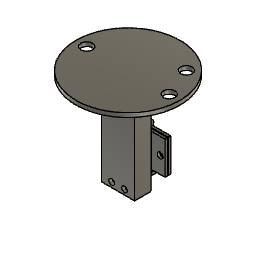
electrode_jig (Autodesk Fusion 360 design; units mm, degrees)
Autodesk Fusion 360 part; units mm, degrees
note: some values were not read from the file. Set by a fixed rule: which sketch regions a step uses.
sketch "スケッチ1" plane through (0, 0, 0) normal (0, 0, 1) x (1, 0, 0)
  circle A0 centre (0, 0) radius 31.5
  circle A1 centre (0, 0) radius 25 construction
  circle A2 centre (-25, 0) radius 3.5
  circle A3 centre (25, 0) radius 3.5
  line L0 (0, 1.75) -> (0, 22.5)
  line L1 (1.75, 0) -> (22.5, 0)
  circle A4 centre (17.6777, 17.6777) radius 3.5
  line L2 (17.6777, 17.6777) -> (0, 0) construction
  dimension "d1" = 63
  dimension "d2" = 50
  dimension "d5" = 7
  dimension "d6" = 7
  dimension "d7" = 7
  dimension "d8" = 45
  constraint coincident A0.centre A1.centre
  constraint coincident A1 A2.centre
  constraint coincident A1 A3.centre
  constraint coincident A3.centre L1
  constraint coincident A2.centre L1
  constraint coincident A1 A4.centre
  constraint coincident A4.centre L2.start
  measures "d1" diameter of A0
  measures "d2" diameter of A1
  measures "d5" diameter of A2
  measures "d6" diameter of A3
  measures "d7" diameter of A4
  measures "d8" angle of L1 L2
extrude "押し出し1" add sketch "スケッチ1" along normal blind 2.5 makes body 1
sketch "スケッチ17" plane through (0, 0, 0) normal (0, 0, -1) x (1, 0, 0)
  circle A0 centre (25, 0) radius 3.5
  circle A1 centre (-25, 0) radius 3.5
  circle A2 centre (17.6777, -17.6777) radius 3.5
  circle A3 centre (0, 0) radius 31.5
  line L0 (10, -4) -> (8, -4)
  line L1 (8, -4) -> (8, 4)
  line L2 (8, 4) -> (-8, 4)
  line L3 (-8, 4) -> (-8, -4)
  line L4 (-8, -4) -> (-10, -4)
  line L5 (-10, -4) -> (-10, 6)
  line L6 (-10, 6) -> (10, 6)
  line L7 (10, 6) -> (10, -4)
  line L8 (8, -4) -> (6, -4)
  line L9 (6, -4) -> (6, -2)
  line L10 (6, -2) -> (8, -2)
  line L11 (8, -2) -> (8, -4)
  line L12 (-8, -4) -> (-6, -4)
  line L13 (-6, -4) -> (-6, -2)
  line L14 (-6, -2) -> (-8, -2)
  line L15 (-8, -2) -> (-8, -4)
  dimension "d138" = 16
  dimension "d139" = 2
  dimension "d140" = 2
  dimension "d142" = 8
  dimension "d143" = 2
  dimension "d144" = 4
  dimension "d145" = 8
  dimension "d178" = 2
  dimension "d179" = 2
  dimension "d180" = 2
  dimension "d181" = 2
  constraint horizontal L0
  constraint perpendicular L0 L1
  constraint perpendicular L1 L2
  constraint perpendicular L2 L3
  constraint perpendicular L1 L4
  constraint perpendicular L4 L5
  constraint perpendicular L1 L6
  constraint perpendicular L6 L7
  constraint collinear L0 L4
  constraint horizontal L8
  constraint vertical L9
  constraint horizontal L10
  constraint vertical L11
  constraint horizontal L12
  constraint vertical L13
  constraint horizontal L14
  constraint vertical L15
  measures "d138" distance of L1.end L2.end
  measures "d139" distance of L3.end L4.end
  measures "d140" distance of L0.start L0.end
  measures "d142" distance of L0.end L1.end
  measures "d143" distance of L2 L6
  measures "d144" distance of A3.centre L2
  measures "d145" distance of A3.centre L3
  measures "d178" distance of L0.end L8.end
  measures "d179" distance of L8.end L9.end
  measures "d180" distance of L3.end L12.end
  measures "d181" distance of L12.end L13.end
extrude "押し出し16" add sketch "スケッチ17" along normal blind 58 contours L0 L1 L2 L3 L4 L5 L6 L7 L11 L15 | L1 L8 L9 L10 L11 | L3 L12 L13 L14 L15 bodies 1
sketch "スケッチ24" plane through (0, 0, 0) normal (0, 0, -1) x (1, 0, 0)
  line L0 (-10, -4) -> (-10, 6)
  line L1 (-10, 6) -> (10, 6)
  line L2 (10, 6) -> (10, -4)
  line L3 (10, -4) -> (6, -4)
  line L4 (6, -4) -> (6, -2)
  line L5 (6, -2) -> (8, -2)
  line L6 (8, -2) -> (8, 4)
  line L7 (8, 4) -> (-8, 4)
  line L8 (-8, 4) -> (-8, -2)
  line L9 (-8, -2) -> (-6, -2)
  line L10 (-6, -2) -> (-6, -4)
  line L11 (-6, -4) -> (-10, -4)
  circle A0 centre (17.6777, -17.6777) radius 3.5
  circle A1 centre (25, 0) radius 3.5
  circle A2 centre (-25, 0) radius 3.5
  circle A3 centre (0, 0) radius 31.5
  line L12 (-10, 6) -> (10, 6)
  line L13 (10, 6) -> (10, -4)
  line L14 (10, -4) -> (-10, -4)
  line L15 (-10, -4) -> (-10, 6)
  constraint horizontal L12
  constraint vertical L13
  constraint horizontal L14
  constraint vertical L15
  constraint coincident L2.end L3.start
  constraint coincident L0.end L1.start
extrude "押し出し24" add sketch "スケッチ24" along normal blind 5 contours L0 L1 L2 L3 L4 L5 L6 L7 L8 L9 L10 L11 L12 L13 L14 L15 | L4 L5 L6 L7 L8 L9 L10 L14 bodies 1
sketch "スケッチ19" plane through (0, 0, 0) normal (0, 0, -1) x (1, 0, 0)
  line L0 (10, 6) -> (10, -4)
  line L1 (10, -4) -> (-10, -4)
  line L2 (-10, -4) -> (-10, 6)
  line L3 (-10, 6) -> (10, 6)
  circle A0 centre (25, 0) radius 3.5
  circle A1 centre (-25, 0) radius 3.5
  circle A2 centre (17.6777, -17.6777) radius 3.5
  circle A3 centre (0, 0) radius 31.5
  circle A4 centre (0, 0) radius 2
  dimension "d152" = 4
  constraint coincident A3.centre A4.centre
  measures "d152" diameter of A4
extrude "押し出し18" add sketch "スケッチ19" along normal blind 50 contours A4 bodies 1
sketch "スケッチ20" plane through (0, 0, -50) normal (0, 0, -1) x (1, 0, 0)
  circle A0 centre (0, 0) radius 2
  line L0 (7.9, -13.5) -> (-7.9, -13.5)
  line L1 (-7.9, -13.5) -> (-7.9, 3.9)
  line L2 (-7.9, 3.9) -> (7.9, 3.9)
  line L3 (7.9, 3.9) -> (7.9, -13.5)
  line L4 (-10, -4) -> (-6, -4)
  line L5 (10, 6) -> (-10, 6)
  line L6 (-10, 6) -> (-10, -4)
  line L7 (-10, -4) -> (-6, -4)
  line L8 (-8, -2) -> (-8, 4)
  line L9 (-8, 4) -> (8, 4)
  line L10 (8, 4) -> (8, -2)
  line L11 (10, -4) -> (10, 6)
  circle A1 centre (0, -8.5) radius 3.25
  line L12 (0, 0) -> (0, -8.5) construction
  line L13 (-6, -4) -> (-6, -2)
  line L14 (-6, -2) -> (-8, -2)
  line L15 (8, -2) -> (6, -2)
  line L16 (6, -2) -> (6, -4)
  line L17 (6, -4) -> (10, -4)
  line L18 (-10, -4) -> (-6, -4)
  line L19 (-6, -4) -> (-6, -2)
  line L20 (-6, -2) -> (-8, -2)
  line L21 (-8, -2) -> (-8, 4)
  line L22 (-8, 4) -> (8, 4)
  line L23 (8, 4) -> (8, -2)
  line L24 (8, -2) -> (6, -2)
  line L25 (6, -2) -> (6, -4)
  line L26 (6, -4) -> (10, -4)
  line L27 (10, -4) -> (10, 6)
  line L28 (10, 6) -> (-10, 6)
  line L29 (-10, 6) -> (-10, -4)
  circle A2 centre (0, 0) radius 2
  line L30 (-7.9, -4.15) -> (-5.8, -4.15)
  line L31 (-5.8, -4.15) -> (-5.8, -1.85)
  line L32 (-5.8, -1.85) -> (-7.9, -1.85)
  line L33 (-7.9, -1.85) -> (-7.9, -4.15)
  line L34 (7.9, -4.15) -> (5.8, -4.15)
  line L35 (5.8, -4.15) -> (5.8, -1.85)
  line L36 (5.8, -1.85) -> (7.9, -1.85)
  line L37 (7.9, -1.85) -> (7.9, -4.15)
  dimension "d155" = 0.1
  dimension "d156" = 0.1
  dimension "d157" = 0.1
  dimension "d173" = 6.5
  dimension "d174" = 5
  dimension "d175" = 8.5
  dimension "d184" = 0.15
  dimension "d185" = 0.15
  dimension "d186" = 0.2
  dimension "d187" = 0.15
  dimension "d188" = 0.15
  dimension "d189" = 0.2
  constraint horizontal L0
  constraint vertical L1
  constraint horizontal L2
  constraint vertical L3
  constraint coincident A0.centre L12.start
  constraint coincident A1.centre L12.end
  constraint perpendicular L2 L12
  constraint coincident L0.end L1.start
  constraint horizontal L30
  constraint vertical L31
  constraint horizontal L32
  constraint vertical L33
  constraint coincident L1 L30.start
  constraint horizontal L34
  constraint vertical L35
  constraint horizontal L36
  constraint vertical L37
  constraint coincident L3 L34.start
  measures "d155" distance of L3 L10
  measures "d156" distance of L2 L9
  measures "d157" distance of L1 L8
  measures "d173" diameter of A1
  measures "d174" distance of L0 A1.centre
  measures "d175" vertical distance of A0.centre A1.centre
  measures "d184" distance of L7 L30
  measures "d185" distance of L20 L32
  measures "d186" distance of L19 L31
  measures "d187" distance of L26 L34
  measures "d188" distance of L15 L36
  measures "d189" distance of L25 L35
extrude "押し出し19" add sketch "スケッチ20" along normal blind 2 separate body contours A0 A2 | L0 L1 L2 L3 L30 L31 L32 L34 L35 L36 makes body 2
sketch "スケッチ21" plane through (0, 0, -52) normal (0, 0, -1) x (1, 0, 0)
  line L0 (7.9, 3.9) -> (-7.9, 3.9)
  line L1 (-7.9, 3.9) -> (-7.9, 1.9)
  line L2 (-7.9, 1.9) -> (7.9, 1.9)
  line L3 (7.9, 1.9) -> (7.9, 3.9)
  line L4 (7.9, 3.9) -> (-7.9, 3.9)
  line L5 (-7.9, 3.9) -> (-7.9, -1.85)
  line L6 (-7.9, -13.5) -> (7.9, -13.5)
  line L7 (7.9, -1.85) -> (7.9, 3.9)
  circle A0 centre (0, -8.5) radius 3.25
  line L8 (7.9, -4.15) -> (5.8, -4.15)
  line L9 (5.8, -4.15) -> (5.8, -1.85)
  line L10 (5.8, -1.85) -> (7.9, -1.85)
  line L11 (-7.9, -1.85) -> (-5.8, -1.85)
  line L12 (-5.8, -1.85) -> (-5.8, -4.15)
  line L13 (-5.8, -4.15) -> (-7.9, -4.15)
  line L14 (-7.9, -4.15) -> (-7.9, -13.5)
  line L15 (7.9, -13.5) -> (7.9, -4.15)
  dimension "d160" = 2
  constraint horizontal L0
  constraint vertical L1
  constraint horizontal L2
  constraint vertical L3
  constraint collinear L0 L4
  measures "d160" distance of L0.start L2.end
extrude "押し出し20" add sketch "スケッチ21" along normal blind 6 contours L0 L1 L2 L3 L4 L5 L7 bodies 2
sketch "スケッチ22" plane through (0, -1.9, 0) normal (0, 1, 0) x (-1, 0, 0)
  line L0 (7.9, -52) -> (-7.9, -52)
  line L1 (-7.9, -52) -> (-7.9, -58)
  line L2 (-7.9, -58) -> (7.9, -58)
  line L3 (7.9, -58) -> (7.9, -52)
  line L4 (-7.9, -55) -> (7.9, -55) construction
  circle A0 centre (-3.9, -55) radius 1.7
  circle A1 centre (3.9, -55) radius 1.7
  dimension "d163" = 3.4
  dimension "d164" = 3.4
  dimension "d166" = 4
  dimension "d167" = 4
  constraint midpoint L1 L4.start
  constraint midpoint L3 L4.end
  constraint coincident L4 A0.centre
  constraint coincident L4 A1.centre
  measures "d163" diameter of A0
  measures "d164" diameter of A1
  measures "d166" distance of L3 A1.centre
  measures "d167" distance of L1 A0.centre
extrude "押し出し21" cut sketch "スケッチ22" against normal up to surface (4.1 mm away) contours A0 | A1 bodies 1 2
ref_plane "作業平面2" through (0, 4.8, -49) normal (0, 0, 1) x (-1, 0, 0)
sketch "スケッチ25" plane through (0, 4.8, -49) normal (0, 0, 1) x (1, 0, 0)
  line L0 (15.9, 3.3) -> (15.9, 1.8)
  line L1 (15.9, 1.8) -> (7.8, 1.8)
  line L2 (5.8, -0.6) -> (5.8, -3)
  line L3 (5.8, -3) -> (7.8, -3)
  line L4 (7.8, -3) -> (7.8, -8.6)
  line L5 (7.8, -8.6) -> (-7.8, -8.6)
  line L6 (-7.8, -8.6) -> (-7.8, -3)
  line L7 (-7.8, -3) -> (-5.8, -3)
  line L8 (-5.8, -3) -> (-5.8, -0.6)
  line L9 (-7.8, 1.8) -> (-15.9, 1.8)
  line L10 (-15.9, 1.8) -> (-15.9, 3.3)
  line L11 (-15.9, 3.3) -> (15.9, 3.3)
  line L12 (-10, -0.8) -> (-6, -0.8)
  line L13 (-6, -0.8) -> (-6, -2.8)
  line L14 (-6, -2.8) -> (-8, -2.8)
  line L15 (-8, -2.8) -> (-8, -8.8)
  line L16 (-8, -8.8) -> (8, -8.8)
  line L17 (8, -8.8) -> (8, -2.8)
  line L18 (8, -2.8) -> (6, -2.8)
  line L19 (6, -2.8) -> (6, -0.8)
  line L20 (6, -0.8) -> (10, -0.8)
  line L21 (10, -0.8) -> (10, -10.8)
  line L22 (10, -10.8) -> (-10, -10.8)
  line L23 (-10, -10.8) -> (-10, -0.8)
  line L24 (-5.8, -0.6) -> (-7.8, -0.6)
  line L25 (-7.8, -0.6) -> (-7.8, 1.8)
  line L26 (7.8, 1.8) -> (7.8, -0.6)
  line L27 (7.8, -0.6) -> (5.8, -0.6)
  line L28 (-15.9, 5.3) -> (-15.9, 3.8)
  line L29 (-15.9, 3.8) -> (15.9, 3.8)
  line L30 (15.9, 3.8) -> (15.9, 5.3)
  line L31 (15.9, 5.3) -> (4.7697, 5.3)
  line L32 (-4.7697, 5.3) -> (-15.9, 5.3)
  arc A0 (4.7697, 5.3) -> (-4.7697, 5.3) centre (0, 3.8) ccw
  circle A1 centre (0, -4.8) radius 2
  circle A2 centre (0, -4.8) radius 2.2
  dimension "d192" = 0.2
  dimension "d193" = 0.2
  dimension "d194" = 0.2
  dimension "d195" = 0.2
  dimension "d196" = 0.2
  dimension "d197" = 0.2
  dimension "d198" = 0.2
  dimension "d199" = 0.2
  dimension "d201" = 0.2
  dimension "d202" = 2
  dimension "d203" = 2
  dimension "d204" = 10.4
  dimension "d205" = 10.4
  dimension "d206" = 1.5
  dimension "d207" = 8.1
  dimension "d208" = 8.1
  dimension "d209" = 1.5
  dimension "d210" = 0.5
  dimension "d211" = 10
  dimension "d214" = 0.2
  constraint vertical L0
  constraint perpendicular L0 L1
  constraint perpendicular L1 L2
  constraint perpendicular L2 L3
  constraint perpendicular L3 L4
  constraint perpendicular L4 L5
  constraint perpendicular L5 L6
  constraint perpendicular L6 L7
  constraint perpendicular L7 L8
  constraint perpendicular L8 L9
  constraint perpendicular L10 L11
  constraint perpendicular L9 L10
  constraint horizontal L24
  constraint vertical L25
  constraint vertical L26
  constraint horizontal L27
  constraint horizontal L31
  constraint vertical L28
  constraint horizontal L29
  constraint vertical L30
  constraint collinear L0 L30
  constraint collinear L10 L28
  constraint midpoint L29 A0.centre
  constraint collinear L31 L32
  constraint concentric A1 A2
  measures "d192" distance of L3 L18
  measures "d193" distance of L4 L17
  measures "d194" distance of L5 L16
  measures "d195" distance of L6 L15
  measures "d196" distance of L7 L14
  measures "d197" distance of L8 L13
  measures "d198" distance of L2 L19
  measures "d199" distance of L20 L27
  measures "d201" distance of L12 L24
  measures "d202" distance of L8.end L24.end
  measures "d203" distance of L26.end L2.start
  measures "d204" distance of L1 L5
  measures "d205" distance of L5 L9
  measures "d206" distance of L0.start L0.end
  measures "d207" distance of L0.end L1.end
  measures "d208" distance of L9.end L9.start
  measures "d209" distance of L30.end L29.end
  measures "d210" distance of L11 L29
  measures "d211" diameter of A0
  measures "d214" distance of A1 A2
extrude "押し出し25" add sketch "スケッチ25" along normal blind 20 separate body contours L0 L1 L2 L3 L4 L5 L6 L7 L8 L9 L10 L11 L24 L25 L26 L27 | L28 L29 L30 L31 L32 A0 makes body 3 at (-5.3, 8.1, -35.6667) makes body 4 at (-5.3, 8.6, -35.6667)
sketch "スケッチ26" plane through (0, 0, -49) normal (0, 0, -1) x (1, 0, 0)
  arc A0 (-4.7697, -10.1) -> (4.7697, -10.1) centre (0, -8.6) ccw
  line L0 (4.7697, -10.1) -> (15.9, -10.1)
  line L1 (15.9, -10.1) -> (15.9, -8.6)
  line L2 (15.9, -8.6) -> (-15.9, -8.6)
  line L3 (-15.9, -8.6) -> (-15.9, -10.1)
  line L4 (-15.9, -10.1) -> (-4.7697, -10.1)
  arc A1 (-2.975, -8.6) -> (2.975, -8.6) centre (0, -8.6) ccw
  circle A2 centre (0, 0) radius 2.2
  line L5 (7.8, -6.6) -> (7.8, -4.2)
  line L6 (7.8, -4.2) -> (5.8, -4.2)
  line L7 (5.8, -4.2) -> (5.8, -1.8)
  line L8 (5.8, -1.8) -> (7.8, -1.8)
  line L9 (7.8, -1.8) -> (7.8, 3.8)
  line L10 (7.8, 3.8) -> (-7.8, 3.8)
  line L11 (-7.8, 3.8) -> (-7.8, -1.8)
  line L12 (-7.8, -1.8) -> (-5.8, -1.8)
  line L13 (-5.8, -1.8) -> (-5.8, -4.2)
  line L14 (-5.8, -4.2) -> (-7.8, -4.2)
  line L15 (-7.8, -4.2) -> (-7.8, -6.6)
  line L16 (-7.8, -6.6) -> (-15.9, -6.6)
  line L17 (-15.9, -6.6) -> (-15.9, -8.1)
  line L18 (-15.9, -8.1) -> (15.9, -8.1)
  line L19 (15.9, -8.1) -> (15.9, -6.6)
  line L20 (15.9, -6.6) -> (7.8, -6.6)
  arc A3 (2.975, -8.1) -> (-2.975, -8.1) centre (0, -8.1) ccw
  dimension "d215" = 5.95
  dimension "d216" = 5.95
  constraint concentric A0 A1
  constraint coincident L2 A1.end
  constraint coincident L2 A1.start
  constraint midpoint L18 A3.centre
  constraint coincident L18 A3.start
  constraint coincident L18 A3.end
  measures "d215" diameter of A1
  measures "d216" diameter of A3
extrude "押し出し26" cut sketch "スケッチ26" against normal blind 18.5 contours L2 A1 | L18 A3 bodies 3 4
sketch "スケッチ27" plane through (0, 0, -29) normal (0, 0, 1) x (-1, 0, 0)
  circle A0 centre (0, 0) radius 2.2
  line L0 (-7.8, -4.2) -> (-7.8, -6.6)
  line L1 (-7.8, -6.6) -> (-15.9, -6.6)
  line L2 (-15.9, -6.6) -> (-15.9, -8.1)
  line L3 (-15.9, -8.1) -> (15.9, -8.1)
  line L4 (15.9, -8.1) -> (15.9, -6.6)
  line L5 (15.9, -6.6) -> (7.8, -6.6)
  line L6 (7.8, -6.6) -> (7.8, -4.2)
  line L7 (7.8, -4.2) -> (5.8, -4.2)
  line L8 (5.8, -4.2) -> (5.8, -1.8)
  line L9 (5.8, -1.8) -> (7.8, -1.8)
  line L10 (7.8, -1.8) -> (7.8, 3.8)
  line L11 (7.8, 3.8) -> (-7.8, 3.8)
  line L12 (-7.8, 3.8) -> (-7.8, -1.8)
  line L13 (-7.8, -1.8) -> (-5.8, -1.8)
  line L14 (-5.8, -1.8) -> (-5.8, -4.2)
  line L15 (-5.8, -4.2) -> (-7.8, -4.2)
  arc A1 (-4.7697, -10.1) -> (4.7697, -10.1) centre (0, -8.6) ccw
  line L16 (4.7697, -10.1) -> (15.9, -10.1)
  line L17 (15.9, -10.1) -> (15.9, -8.6)
  line L18 (15.9, -8.6) -> (-15.9, -8.6)
  line L19 (-15.9, -8.6) -> (-15.9, -10.1)
  line L20 (-15.9, -10.1) -> (-4.7697, -10.1)
  arc A2 (1.125, -8.1) -> (-1.125, -8.1) centre (0, -8.1) ccw
  arc A3 (-1.125, -8.6) -> (1.125, -8.6) centre (0, -8.6) ccw
  dimension "d219" = 2.25
  dimension "d220" = 2.25
  constraint midpoint L3 A2.centre
  constraint coincident L3 A2.start
  constraint coincident L3 A2.end
  constraint concentric A1 A3
  constraint coincident L18 A3.end
  constraint coincident L18 A3.start
  measures "d219" diameter of A2
  measures "d220" diameter of A3
extrude "押し出し27" cut sketch "スケッチ27" against normal blind 1.5 contours L3 A2 | L18 A3 bodies 3 4
sketch "スケッチ28" plane through (0, 0, -29) normal (0, 0, 1) x (-1, 0, 0)
  arc A0 (1.125, -8.1) -> (-1.125, -8.1) centre (0, -8.1) ccw
  line L0 (1.125, -8.1) -> (15.9, -8.1)
  line L1 (15.9, -8.1) -> (15.9, -6.6)
  line L2 (15.9, -6.6) -> (7.8, -6.6)
  line L3 (7.8, -6.6) -> (7.8, -4.2)
  line L4 (7.8, -4.2) -> (5.8, -4.2)
  line L5 (5.8, -4.2) -> (5.8, -1.8)
  line L6 (5.8, -1.8) -> (7.8, -1.8)
  line L7 (7.8, -1.8) -> (7.8, 3.8)
  line L8 (7.8, 3.8) -> (-7.8, 3.8)
  line L9 (-7.8, 3.8) -> (-7.8, -1.8)
  line L10 (-7.8, -1.8) -> (-5.8, -1.8)
  line L11 (-5.8, -1.8) -> (-5.8, -4.2)
  line L12 (-5.8, -4.2) -> (-7.8, -4.2)
  line L13 (-7.8, -4.2) -> (-7.8, -6.6)
  line L14 (-7.8, -6.6) -> (-15.9, -6.6)
  line L15 (-15.9, -6.6) -> (-15.9, -8.1)
  line L16 (-15.9, -8.1) -> (-1.125, -8.1)
  circle A1 centre (0, 0) radius 2.2
  circle A2 centre (0, 0) radius 3
  dimension "d223" = 6
  constraint concentric A1 A2
  measures "d223" diameter of A2
extrude "押し出し28" cut sketch "スケッチ28" against normal blind 2 contours A2 bodies 3
sketch "スケッチ29" plane through (0, 10.1, 0) normal (0, 1, 0) x (-1, 0, 0)
  line L0 (-15.9, -49) -> (-4.7697, -49)
  line L1 (-4.7697, -49) -> (-4.7697, -29)
  line L2 (-4.7697, -29) -> (-15.9, -29)
  line L3 (-15.9, -29) -> (-15.9, -49)
  line L4 (-12.9, -29) -> (-12.9, -49) construction
  line L5 (12.9, -29) -> (12.9, -49) construction
  line L6 (15.9, -49) -> (15.9, -29) construction
  circle A0 centre (-12.9, -39) radius 1.75
  circle A1 centre (12.9, -39) radius 1.75
  line L7 (4.7697, -29) -> (15.9, -29)
  line L8 (4.7697, -49) -> (15.9, -49)
  dimension "d226" = 3
  dimension "d227" = 3
  dimension "d228" = 3.5
  dimension "d229" = 3.5
  constraint coincident L2 L4.start
  constraint coincident L0 L4.end
  constraint perpendicular L0 L4
  constraint perpendicular L0 L5
  constraint midpoint L4 A0.centre
  constraint midpoint L5 A1.centre
  constraint coincident L5.start L7
  constraint coincident L5.end L8
  measures "d226" distance of L3 L4
  measures "d227" distance of L5 L6
  measures "d228" diameter of A0
  measures "d229" diameter of A1
extrude "押し出し29" cut sketch "スケッチ29" against normal up to surface (3.5 mm away) contours A0 | A1 bodies 3 4
component "Component" placed x (1, 0, 0) y (0, 1, 0) z (0, 0, 1) at (0, 0, 0)
